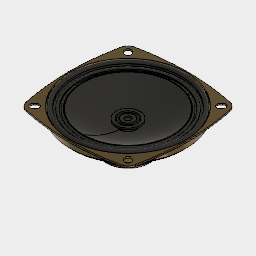
1313 Speaker 3in 8Ohm 1W (Autodesk Fusion 360 design; units mm, degrees)
Autodesk Fusion 360 part; units mm, degrees
sketch "frame" plane through (0, 0, 0) normal (0, 0, 1) x (1, 0, 0)
  circle A0 centre (0, 0) radius 38.1
  line L0 (38.9, -38.9) -> (-38.9, -38.9)
  line L1 (-38.9, -38.9) -> (-38.9, 38.9)
  line L2 (-38.9, 38.9) -> (38.9, 38.9)
  line L3 (38.9, 38.9) -> (38.9, -38.9)
  line L4 (38.9, -38.9) -> (-38.9, 38.9) construction
  line L5 (-38.9, -38.9) -> (38.9, 38.9) construction
  spline S0 degree 5 poles (-38.9, 33.9) (-37.344, 34.2792) (-34.232, 35.0046) (-29.564, 35.9933) (-23.34, 37.1095) (-15.56, 38.1453) (-7.78, 38.7894) (0, 39.01) (7.78, 38.7894) (15.56, 38.1453) (23.34, 37.1095) (29.564, 35.9933) (34.232, 35.0046) (37.344, 34.2792) (38.9, 33.9) knots 0 0 0 0 0 0 0.1 0.2 0.3 0.4 0.5 0.6 0.7 0.8 0.9 1 1 1 1 1 1
  spline S1 degree 5 poles (-33.9, -38.9) (-34.2792, -37.344) (-35.0046, -34.232) (-35.9933, -29.564) (-37.1095, -23.34) (-38.1453, -15.56) (-38.7894, -7.78) (-39.01, 0) (-38.7894, 7.78) (-38.1453, 15.56) (-37.1095, 23.34) (-35.9933, 29.564) (-35.0046, 34.232) (-34.2792, 37.344) (-33.9, 38.9) knots 0 0 0 0 0 0 0.1 0.2 0.3 0.4 0.5 0.6 0.7 0.8 0.9 1 1 1 1 1 1
  spline S2 degree 5 poles (38.9, -33.9) (37.344, -34.2792) (34.232, -35.0046) (29.564, -35.9933) (23.34, -37.1095) (15.56, -38.1453) (7.78, -38.7894) (0, -39.01) (-7.78, -38.7894) (-15.56, -38.1453) (-23.34, -37.1095) (-29.564, -35.9933) (-34.232, -35.0046) (-37.344, -34.2792) (-38.9, -33.9) knots 0 0 0 0 0 0 0.1 0.2 0.3 0.4 0.5 0.6 0.7 0.8 0.9 1 1 1 1 1 1
  spline S3 degree 5 poles (33.9, 38.9) (34.2792, 37.344) (35.0046, 34.232) (35.9933, 29.564) (37.1095, 23.34) (38.1453, 15.56) (38.7894, 7.78) (39.01, 0) (38.7894, -7.78) (38.1453, -15.56) (37.1095, -23.34) (35.9933, -29.564) (35.0046, -34.232) (34.2792, -37.344) (33.9, -38.9) knots 0 0 0 0 0 0 0.1 0.2 0.3 0.4 0.5 0.6 0.7 0.8 0.9 1 1 1 1 1 1
  line L6 (-32.4142, 29.5858) -> (-31.4243, 28.5958)
  arc A1 (-31.4243, 28.5958) -> (-28.5958, 31.4243) centre (-30.0101, 30.0101) ccw
  line L7 (-28.5958, 31.4243) -> (-29.5858, 32.4142)
  arc A2 (-29.5858, 32.4142) -> (-32.4142, 29.5858) centre (-31, 31) ccw
  line L8 (-31, 31) -> (-30.0101, 30.0101) construction
  arc A3 (-28.5958, -31.4243) -> (-31.4243, -28.5958) centre (-30.0101, -30.0101) ccw
  line L9 (-31.4243, -28.5958) -> (-32.4142, -29.5858)
  line L10 (-29.5858, -32.4142) -> (-28.5958, -31.4243)
  arc A4 (-32.4142, -29.5858) -> (-29.5858, -32.4142) centre (-31, -31) ccw
  arc A5 (31.4243, -28.5958) -> (28.5958, -31.4243) centre (30.0101, -30.0101) ccw
  line L11 (28.5958, -31.4243) -> (29.5858, -32.4142)
  line L12 (32.4142, -29.5858) -> (31.4243, -28.5958)
  arc A6 (29.5858, -32.4142) -> (32.4142, -29.5858) centre (31, -31) ccw
  arc A7 (28.5958, 31.4243) -> (31.4243, 28.5958) centre (30.0101, 30.0101) ccw
  line L13 (31.4243, 28.5958) -> (32.4142, 29.5858)
  line L14 (29.5858, 32.4142) -> (28.5958, 31.4243)
  arc A8 (32.4142, 29.5858) -> (29.5858, 32.4142) centre (31, 31) ccw
  point P0 (0, 38.9)
  point P1 (-38.9, 0)
  point P2 (0, -38.9)
  point P3 (38.9, 0)
  dimension "d1" = 76.2
  dimension "d2" = 77.8
  dimension "d3" = 77.8
  dimension "d4" = 5
  dimension "d5" = 5
  dimension "d7" = 360
  dimension "d11" = 4
  dimension "d13" = 360
  dimension "d30" = 1.4
  measures "d1" diameter of A0
  measures "d2" distance of L1.end L2.end
  measures "d3" distance of L0.end L1.end
  measures "d4" distance of L1.end S0.start
  measures "d5" distance of L2.end S0.end
  measures "d11" diameter of A1
  measures "d30" distance of A2.centre A1.centre
extrude "Extrude1" add sketch "frame" along normal blind 1 contours S0 S1 S2 S3 makes body 1
fillet "Fillet1" radius 6 4 edges at (-34.8436, -34.8436, 0.5) (-34.8436, 34.8436, 0.5) (34.8436, -34.8436, 0.5) (34.8436, 34.8436, 0.5) on bodies 1
sketch "circle" plane through (0, 0, 0) normal (0, 0, 1) x (1, 0, 0)
  circle A0 centre (0, 0) radius 38.1
  dimension "d14" = 76.2
  measures "d14" diameter of A0
sketch "cone" plane through (0, 0, 0) normal (1, 0, 0) x (0, 1, 0)
  line L0 (38.1, 0) -> (-38.1, 0) construction
  line L1 (-37.5, 0) -> (-37.5, 1.5)
  line L2 (-37.5, 1.5) -> (-34.9, 1.5)
  line L3 (-34.9, 1.5) -> (-34.9, -1)
  line L4 (-34.9, -1) -> (-33.4, -1)
  line L5 (-33.4, -1) -> (-33.4, 0)
  line L6 (-31.9, 0) -> (-31.9, -1.5)
  line L7 (-31.9, -1.5) -> (-30.9, -1.5)
  line L8 (-30.9, -1.5) -> (-30.9, -0.5)
  line L9 (-30.9, -0.5) -> (-29.4, -0.5)
  line L10 (0, 0) -> (0, -10) construction
  spline S0 degree 5 poles (-29.4, -0.5) (-28.4466, -1.0907) (-26.514, -2.2477) (-23.5375, -3.9098) (-19.4028, -5.9686) (-13.8223, -8.1522) (-8.8206, -9.3903) (-4.6152, -9.8891) (-1.5774, -10) (0, -10) knots 0 0 0 0 0 0 0.2 0.4 0.6 0.8 1 1 1 1 1 1
  line L11 (-4, -10) -> (4, -10)
  line L12 (-37.5, 0) -> (-37.5, -13)
  line L13 (-37.5, -13) -> (0, -13)
  line L14 (0, -13) -> (0, -10)
  line L15 (-33.4, 0) -> (-31.9, 0)
  spline S1 degree 5 poles (0, -13) (-1.5762, -13) (-4.7064, -12.8728) (-9.335, -12.3006) (-15.3915, -10.8801) (-22.8346, -8.3751) (-28.7266, -6.0131) (-33.1219, -4.1064) (-36.0423, -2.7791) (-37.5, -2.1014) knots 0 0 0 0 0 0 0.2 0.4 0.6 0.8 1 1 1 1 1 1
  line L16 (4, -13) -> (-4, -13)
  dimension "d19" = 1
  dimension "d20" = 1.5
  dimension "d21" = 1.5
  dimension "d22" = 1
  dimension "d23" = 1.5
  dimension "d24" = 1
  dimension "d25" = 1.5
  dimension "d26" = 2.5
  dimension "d27" = 2.6
  dimension "d28" = 10
  dimension "d29" = 3
  measures "d19" distance of L7.end L8.end
  measures "d20" distance of L8.end L9.end
  measures "d21" distance of L6.start L6.end
  measures "d22" distance of L6.end L7.end
  measures "d23" distance of L5.end L6.start
  measures "d24" distance of L4.end L5.end
  measures "d25" distance of L3.end L4.end
  measures "d26" distance of L2.end L3.end
  measures "d27" distance of L1.end L2.end
  measures "d28" distance of L10.start L10.end
  measures "d29" distance of L10.end L13.end
revolve "Revolve1" add sketch "cone" angle 360 about axis through (0, 0, 0) along (0, 0, -1) separate body contours L1 L2 L3 L4 L5 L6 L7 L8 L9 S0 L12 L14 L15 S1 makes body 2
fillet "Fillet2" radius 1.3 2 edges at (-34.9623, -13.5606, 1.5) (-32.5382, -12.6204, 1.5) on bodies 2
fillet "Fillet3" radius 0.75 2 edges at (-31.1397, -12.078, 0) (-29.7412, -11.5355, 0) on bodies 2
fillet "Fillet4" radius 1 1 edges at (-28.8089, -11.1739, -0.5) on bodies 2
sketch "center" plane through (0, 0, 0) normal (0, 0, 1) x (1, 0, 0)
  circle A0 centre (0, 0) radius 7.9
  circle A1 centre (0, 0) radius 4.5
  circle A2 centre (0, 0) radius 1.5
  circle A3 centre (0, 0) radius 5.5
  dimension "d31" = 15.8
  dimension "d32" = 9
  dimension "d33" = 3
  dimension "d34" = 1
  measures "d31" diameter of A0
  measures "d32" diameter of A1
  measures "d33" diameter of A2
extrude "Extrude2" add sketch "center" against normal blind 1 from surface at -6 separate body contours A0 | A1 | A2 | A3 makes body 3
extrude "Extrude3" cut sketch "center" against normal blind 0.5 from surface at -6 contours A2 | A3 bodies 3
fillet "Fillet5" radius 0.5 3 edges at (-5.1278, 1.9889, -6) (-4.1955, -1.6273, -6) (-1.3985, 0.5424, -6) on bodies 3
sketch "container" plane through (0, 0, 0) normal (1, 0, 0) x (0, 1, 0)
  line L0 (-38.1, 0) -> (38.1, 0)
  line L1 (-38.1, 0) -> (-38.1, -4)
  line L2 (-38.1, -4) -> (-36.1, -4)
  line L3 (-36.1, -4) -> (-36.1, -6)
  line L4 (-36.1, -6) -> (-20, -11)
  line L5 (0, 0) -> (0, -24.5)
  line L6 (-20, -11) -> (-17, -14)
  line L7 (-17, -14) -> (-14, -14)
  line L8 (-14, -14) -> (-14, -16)
  line L9 (-14, -16) -> (-16, -16)
  line L10 (-16, -16) -> (-16, -22)
  line L11 (-16, -22) -> (-14, -22)
  line L12 (-14, -22) -> (-14, -24.5)
  line L13 (-14, -24.5) -> (0, -24.5)
  line L14 (-37.1, 0) -> (-37.1, -3)
  line L15 (-37.1, -3) -> (-35.1, -3)
  line L16 (-35.1, -3) -> (-35.1, -5.2634)
  line L17 (-35.1, -5.2634) -> (-19.4675, -10.1182)
  line L18 (-19.4675, -10.1182) -> (-16.5858, -13)
  line L19 (-16.5858, -13) -> (0, -13)
  dimension "d42" = 20
  dimension "d44" = 2
  dimension "d45" = 2
  dimension "d46" = 4
  dimension "d47" = 5
  dimension "d48" = 17
  dimension "d50" = 2
  dimension "d51" = 6
  dimension "d52" = 24.5
  dimension "d66" = 16
  dimension "d67" = 14
  dimension "d69" = 14
  measures "d42" distance of L4.end L5
  measures "d44" distance of L1.end L2.end
  measures "d45" distance of L2.end L3.end
  measures "d46" distance of L0.start L1.end
  measures "d47" distance of L3.end L4.end
  measures "d48" distance of L5 L6.end
  measures "d50" distance of L7.end L8.end
  measures "d51" distance of L9.end L10.end
  measures "d52" distance of L5.start L5.end
  measures "d66" distance of L5 L10
  measures "d67" distance of L5 L12
  measures "d69" distance of L5 L8
revolve "Revolve2" add sketch "container" angle 360 about axis through (0, 0, 0) along (0, 0, -1) separate body contours L0 L1 L2 L3 L4 L5 L6 L7 L8 L9 L10 L11 L12 L13 L14 L15 L16 L17 L18 L19 makes body 4
sketch "Sketch6" plane through (0, 0, 0) normal (0, 0, 1) x (1, 0, 0)
  line L0 (-40, -5) -> (40, -5)
  line L1 (40, -5) -> (40, 5)
  line L2 (40, 5) -> (-40, 5)
  line L3 (-40, 5) -> (-40, -5)
  line L4 (-40, -5) -> (40, 5) construction
  line L5 (40, -5) -> (-40, 5) construction
  line L6 (5, 40) -> (-5, 40)
  line L7 (-5, 40) -> (-5, -40)
  line L8 (-5, -40) -> (5, -40)
  line L9 (5, -40) -> (5, 40)
  line L10 (5, 40) -> (-5, -40) construction
  line L11 (-5, 40) -> (5, -40) construction
  circle A0 centre (0, 0) radius 32
  circle A1 centre (0, 0) radius 20
  dimension "d55" = 10
  dimension "d56" = 80
  dimension "d57" = 80
  dimension "d58" = 10
  dimension "d59" = 64
  measures "d55" distance of L0.end L1.end
  measures "d56" distance of L1.end L2.end
  measures "d57" distance of L6.end L7.end
  measures "d58" distance of L7.end L8.end
  measures "d59" diameter of A0
extrude "Extrude4" cut sketch "Sketch6" against normal blind 30 contours L0 L7 A0 A1 | L2 L7 A0 A1 | L0 L9 A0 A1 | L2 L9 A0 A1 bodies 4
fillet "Fillet6" radius 2 15 edges at (-5, -19.3649, -10.4764) (-5, -31.607, -6.7497) (5, -31.607, -6.7497) (-19.3649, -5, -10.4764) (-31.607, -5, -6.7497) (-31.607, 5, -6.7497) (-5, 19.3649, -10.4764) (-5, 31.607, -6.7497) (5, 31.607, -6.7497) (5, 19.3649, -10.4764) (19.3649, 5, -10.4764) (31.607, 5, -6.7497) (31.607, -5, -6.7497) (19.3649, -5, -10.4764) (-19.3649, 5, -10.4764) on bodies 4
extrude "Extrude5" add sketch "center" against normal blind 3 from surface at -7 contours A1 | A2 | A3 bodies 2 3
equation "d66 = ( 32 / 2 ) * 1 mm"
named bodies: "frame", "cone", "center", "container"
